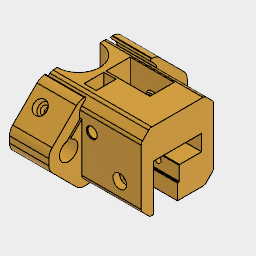
Y_Carriage_1.0_F01 (Autodesk Fusion 360 design; units mm, degrees)
Autodesk Fusion 360 part; units mm, degrees
sketch "スケッチ1" plane through (0, 0, 0) normal (1, 0, 0) x (0, 1, 0)
  line L0 (-17.5, 17.5) -> (17.5, 17.5)
  line L1 (17.5, 17.5) -> (31.5, 3.5)
  line L2 (31.5, 3.5) -> (31.5, -3.5)
  line L3 (31.5, -3.5) -> (17.5, -17.5)
  line L4 (17.5, -17.5) -> (-17.5, -17.5)
  line L5 (-17.5, -17.5) -> (-31.5, -3.5)
  line L6 (-31.5, -3.5) -> (-31.5, 3.5)
  line L7 (-31.5, 3.5) -> (-17.5, 17.5)
  circle A0 centre (-22.5, 0) radius 4.2
  circle A1 centre (22.5, 0) radius 4.2
  line L8 (-12.5, 17.5) -> (-16.5, 13.5)
  line L9 (-16.5, 13.5) -> (-16.5, -13.5)
  line L10 (-16.5, -13.5) -> (-12.5, -17.5)
  line L11 (12.5, 17.5) -> (16.5, 13.5)
  line L12 (16.5, 13.5) -> (16.5, -13.5)
  line L13 (16.5, -13.5) -> (12.5, -17.5)
  line L14 (-13.9142, 17.5) -> (-17.5, 13.9142)
  line L15 (-17.5, 13.9142) -> (-17.5, 9.9071)
  line L16 (-17.5, 9.9071) -> (-23.2802, 4.1269)
  line L17 (-21.8444, 4.1485) -> (-16.5, 9.4929)
  line L18 (-22.5, 0) -> (-22.5, 4.2) construction
  line L19 (-22.5, 4.2) -> (-16.5, 10.2) construction
  line L20 (-22.5, 4.2) -> (-14.0147, 4.2) construction
  line L21 (0, 17.5) -> (0, -17.5) construction
  line L22 (17.5, 9.9071) -> (23.2802, 4.1269)
  line L23 (21.8444, 4.1485) -> (16.5, 9.4929)
  line L24 (17.5, 13.9142) -> (17.5, 9.9071)
  line L25 (13.9142, 17.5) -> (17.5, 13.9142)
  line L26 (12.5, 17.5) -> (16.5, 13.5)
  dimension "d1" = 35
  dimension "d2" = 17.5
  dimension "d3" = 63
  dimension "d4" = 31.5
  dimension "d5" = 14
  dimension "d6" = 14
  dimension "d7" = 14
  dimension "d8" = 14
  dimension "d9" = 14
  dimension "d10" = 14
  dimension "d11" = 14
  dimension "d12" = 14
  dimension "d13" = 8.4
  dimension "d14" = 8.4
  dimension "d15" = 9
  dimension "d16" = 9
  dimension "d17" = 17.5
  dimension "d18" = 17.5
  dimension "d19" = 4
  dimension "d20" = 4
  dimension "d21" = 4
  dimension "d22" = 4
  dimension "d23" = 4
  dimension "d24" = 4
  dimension "d25" = 4
  dimension "d26" = 4
  dimension "d27" = 33
  dimension "d28" = 16.5
  dimension "d29" = 1
  dimension "d30" = 1
  dimension "d31" = 1
  dimension "d32" = 45
  dimension "d33" = 0.5
  measures "d1" distance of L0 L4
  measures "d2" distance of origin L0
  measures "d3" distance of L2 L6
  measures "d4" distance of origin L6
  measures "d5" distance of L0.end L2
  measures "d6" distance of L2.end L3.end
  measures "d7" distance of L0.start L6.end
  measures "d8" distance of L4.end L5.end
  measures "d9" distance of L0.end L1.end
  measures "d10" distance of L2.end L3.end
  measures "d11" distance of L0.start L6.end
  measures "d12" distance of L4.end L5.end
  measures "d13" diameter of A0
  measures "d14" diameter of A1
  measures "d15" distance of L6 A0.centre
  measures "d16" distance of L2 A1.centre
  measures "d17" distance of L0 A0.centre
  measures "d18" distance of L0 A1.centre
  measures "d19" distance of L8.start L8.end
  measures "d20" distance of L11.start L11.end
  measures "d21" distance of L12.end L13.end
  measures "d22" distance of L9.end L10.end
  measures "d23" distance of L8.start L8.end
  measures "d24" distance of L11.start L11.end
  measures "d25" distance of L12.end L13.end
  measures "d26" distance of L9.end L10.end
  measures "d27" distance of L9 L12
  measures "d28" distance of origin L9
  measures "d29" distance of L8 L14
  measures "d30" distance of L9 L15
  measures "d31" distance of L16 L17
  measures "d32" angle of L19 L20
  measures "d33" distance of L17 L19
extrude "押し出し1" add sketch "スケッチ1" along normal blind 45 contours L0 L4 L8 L9 L10 L11 L12 L13 L26
extrude "押し出し2" add sketch "スケッチ1" along normal blind 18 contours L0 L4 L5 L6 L7 A0 L9 L10 L14 L15 L16 L17 | L0 L1 L2 L3 L4 A1 L12 L13 L22 L23 L24 L25
sketch "スケッチ2" plane through (0, 0, 17.5) normal (0, 0, 1) x (-1, 0, 0)
  line L0 (0, -12.5) -> (0, 12.5)
  line L1 (0, 12.5) -> (-45, 12.5)
  line L2 (-45, 12.5) -> (-45, -12.5)
  line L3 (-45, -12.5) -> (0, -12.5)
  line L4 (-12.5, -11) -> (-32.5, -11)
  line L5 (-32.5, -11) -> (-32.5, 0)
  line L6 (-32.5, 0) -> (-12.5, 0)
  line L7 (-12.5, 0) -> (-12.5, -11)
  line L8 (-12.5, 1) -> (-18, 1)
  line L9 (-18, 1) -> (-18, 10)
  line L10 (-18, 10) -> (-12.5, 10)
  line L11 (-12.5, 10) -> (-12.5, 1)
  circle A0 centre (0, 0) radius 9.7
  line L12 (0, -16.5) -> (-45, -16.5)
  line L13 (0, 16.5) -> (-45, 16.5)
  dimension "d38" = 19.4
  dimension "d39" = 32.5
  dimension "d40" = 5.5
  dimension "d41" = 32.5
  dimension "d42" = 20
  dimension "d43" = 11
  dimension "d44" = 9
  dimension "d45" = 5.5
  dimension "d46" = 6.5
  measures "d38" diameter of A0
  measures "d39" distance of L2 L11
  measures "d40" distance of L9 L11
  measures "d41" distance of L2 L7
  measures "d42" distance of L5 L7
  measures "d43" distance of L4 L6
  measures "d44" distance of L8 L10
  measures "d45" distance of L4 L12
  measures "d46" distance of L10 L13
extrude "押し出し3" cut sketch "スケッチ2" against normal up to surface (35 mm away) contours L0 A0 picked at (-3.2243, 0.2416)
sketch "スケッチ3" plane through (45, 0, 0) normal (1, 0, 0) x (0, 1, 0)
  line L0 (-12.5, 17.5) -> (-16.5, 13.5)
  line L1 (-16.5, 13.5) -> (-16.5, -13.5)
  line L2 (-16.5, -13.5) -> (-12.5, -17.5)
  line L3 (-12.5, -17.5) -> (12.5, -17.5)
  line L4 (12.5, -17.5) -> (16.5, -13.5)
  line L5 (16.5, -13.5) -> (16.5, 13.5)
  line L6 (16.5, 13.5) -> (12.5, 17.5)
  line L7 (12.5, 17.5) -> (-12.5, 17.5)
  line L8 (-11, 3.635) -> (0, 3.635)
  line L9 (0, 3.635) -> (0, -17.5)
  line L10 (0, -17.5) -> (-11, -17.5)
  line L11 (-11, -17.5) -> (-11, 3.635)
  line L12 (0, 3.635) -> (11, 3.635)
  line L13 (11, 3.635) -> (11, -3.635)
  line L14 (11, -3.635) -> (0, -3.635)
  line L15 (0, -3.635) -> (0, 3.635)
  dimension "d49" = 5.5
  dimension "d50" = 11
  dimension "d51" = 11
  dimension "d52" = 21.135
  dimension "d53" = 7.27
  measures "d49" distance of L1 L11
  measures "d50" distance of L9 L11
  measures "d51" distance of L9 L13
  measures "d52" distance of L8 L10
  measures "d53" distance of L12 L14
extrude "押し出し4" cut sketch "スケッチ3" against normal blind 19.77 contours L3 L8 L9 L10 L11 L15
fillet "フィレット1" radius 10 1 edges at (25.23, -5.5, 3.635)
extrude "押し出し5" cut sketch "スケッチ2" against normal blind 21.135 contours L4 L5 L6 L7
extrude "押し出し6" cut sketch "スケッチ3" against normal up to surface (12.5 mm away) contours L9 L12 L13 L14 L15
extrude "押し出し7" cut sketch "スケッチ2" against normal up to surface (35 mm away) contours L8 L9 L10 L11
fillet "フィレット2" radius 10 1 edges at (12.5, 5.5, -3.635)
sketch "スケッチ4" plane through (0, 0, 0) normal (0, -1, 0) x (1, 0, 0)
  line L0 (45, -3.635) -> (25.6099, -3.635)
  arc A0 (25.6099, -3.635) -> (25.23, -6.365) centre (35.23, -6.365) ccw
  line L1 (25.23, -6.365) -> (25.23, -17.5)
  line L2 (25.23, -17.5) -> (45, -17.5)
  line L3 (45, -17.5) -> (45, -3.635)
  line L4 (45, -3.635) -> (31, -3.635)
  line L5 (31, -3.635) -> (31, -10.45)
  line L6 (31, -10.45) -> (45, -10.45)
  line L7 (45, -10.45) -> (45, -3.635)
  dimension "d64" = 6.815
  dimension "d65" = 14
  measures "d64" distance of L4 L6
  measures "d65" distance of L5 L7
extrude "押し出し8" cut sketch "スケッチ4" against normal blind 0.8 contours L0 L3 L4 L5 L6 L7
sketch "スケッチ5" plane through (0, -16.5, 0) normal (0, -1, 0) x (1, 0, 0)
  line L0 (0, 9.4929) -> (18, 9.4929)
  line L1 (18, 9.4929) -> (18, -13.5)
  line L2 (18, -13.5) -> (45, -13.5)
  line L3 (45, -13.5) -> (45, 13.5)
  line L4 (45, 13.5) -> (0, 13.5)
  line L5 (0, 13.5) -> (0, 9.4929)
  circle A0 centre (35.23, -6.365) radius 1.5
  circle A1 centre (35.23, -6.365) radius 3.1
  line L6 (18, -17.5) -> (45, -17.5)
  dimension "d68" = 3
  dimension "d69" = 6.2
  dimension "d70" = 9.77
  dimension "d71" = 11.135
  measures "d68" diameter of A0
  measures "d69" diameter of A1
  measures "d70" distance of L3 A0.centre
  measures "d71" distance of A0.centre L6
extrude "押し出し9" cut sketch "スケッチ5" against normal up to surface (33 mm away) contours A0
extrude "押し出し10" cut sketch "スケッチ5" against normal blind 3 contours A1
sketch "スケッチ6" plane through (0, 16.5, 0) normal (0, 1, 0) x (-1, 0, 0)
  circle A0 centre (-35.23, -6.365) radius 1.5
  line L0 (-18, 9.4929) -> (0, 9.4929)
  line L1 (0, 9.4929) -> (0, 13.5)
  line L2 (0, 13.5) -> (-45, 13.5)
  line L3 (-45, 13.5) -> (-45, -13.5)
  line L4 (-45, -13.5) -> (-18, -13.5)
  line L5 (-18, -13.5) -> (-18, 9.4929)
  circle A1 centre (-35.23, -6.365) radius 2.5
  circle A2 centre (-35.23, -6.365) radius 2.25
  circle A3 centre (-22.5, 6.365) radius 1.5
  circle A4 centre (-22.5, 6.365) radius 3.1
  line L6 (0, 17.5) -> (-45, 17.5)
  dimension "d76" = 5
  dimension "d77" = 4.5
  dimension "d82" = 3
  dimension "d83" = 6.2
  dimension "d88" = 11.135
  dimension "d89" = 22.5
  measures "d76" diameter of A1
  measures "d77" diameter of A2
  measures "d82" diameter of A3
  measures "d83" diameter of A4
  measures "d88" distance of A3.centre L6
  measures "d89" distance of L3 A3.centre
extrude "押し出し11" cut sketch "スケッチ6" against normal blind 5 contours A2
extrude "押し出し12" cut sketch "スケッチ6" against normal blind 0.5 contours A1
extrude "押し出し13" cut sketch "スケッチ6" against normal up to surface (33 mm away) contours A3
extrude "押し出し14" cut sketch "スケッチ6" against normal blind 3 contours A4
sketch "スケッチ7" plane through (0, -16.5, 0) normal (0, -1, 0) x (1, 0, 0)
  circle A0 centre (22.5, 6.365) radius 1.5
  circle A1 centre (35.23, -6.365) radius 3.1
  line L0 (0, 9.4929) -> (18, 9.4929)
  line L1 (18, 9.4929) -> (18, -13.5)
  line L2 (18, -13.5) -> (45, -13.5)
  line L3 (45, -13.5) -> (45, 13.5)
  line L4 (45, 13.5) -> (0, 13.5)
  line L5 (0, 13.5) -> (0, 9.4929)
  circle A2 centre (22.5, 6.365) radius 2.5
  circle A3 centre (22.5, 6.365) radius 2.25
  dimension "d90" = 5
  dimension "d91" = 4.5
  measures "d90" diameter of A2
  measures "d91" diameter of A3
extrude "押し出し15" cut sketch "スケッチ7" against normal blind 5 contours A3
extrude "押し出し16" cut sketch "スケッチ7" against normal blind 0.5 contours A2
sketch "スケッチ8" plane through (0, -11, 0) normal (0, 1, 0) x (-1, 0, 0)
  circle A0 centre (-35.23, -6.365) radius 1.5
  arc A1 (-25.23, -6.365) -> (-35.23, 3.635) centre (-35.23, -6.365) ccw
  line L0 (-35.23, 3.635) -> (-45, 3.635)
  line L1 (-45, 3.635) -> (-45, -17.5)
  line L2 (-45, -17.5) -> (-25.23, -17.5)
  line L3 (-25.23, -17.5) -> (-25.23, -6.365)
  circle A2 centre (-35.23, -6.365) radius 2.75
  dimension "d96" = 5.5
  measures "d96" diameter of A2
sketch "スケッチ9" plane through (0, 11, 0) normal (0, -1, 0) x (1, 0, 0)
  circle A0 centre (22.5, 6.365) radius 1.5
  arc A1 (12.5, 6.365) -> (22.5, -3.635) centre (22.5, 6.365) ccw
  line L0 (22.5, -3.635) -> (45, -3.635)
  line L1 (45, -3.635) -> (45, 3.635)
  line L2 (45, 3.635) -> (32.5, 3.635)
  line L3 (32.5, 3.635) -> (32.5, 17.5)
  line L4 (32.5, 17.5) -> (12.5, 17.5)
  line L5 (12.5, 17.5) -> (12.5, 6.365)
  circle A2 centre (22.5, 6.365) radius 2.75
  dimension "d101" = 5.5
  measures "d101" diameter of A2
sketch "スケッチ10" plane through (0, 0, 0) normal (0, 1, 0) x (-1, 0, 0)
  circle A0 centre (-22.5, 6.365) radius 1.5
  arc A1 (-22.5, -3.635) -> (-12.5, 6.365) centre (-22.5, 6.365) ccw
  line L0 (-12.5, 6.365) -> (-12.5, 17.5)
  line L1 (-12.5, 17.5) -> (-32.5, 17.5)
  line L2 (-32.5, 17.5) -> (-32.5, 3.635)
  line L3 (-32.5, 3.635) -> (-35.23, 3.635)
  arc A2 (-25.6099, -3.635) -> (-35.23, 3.635) centre (-35.23, -6.365) ccw
  line L4 (-25.6099, -3.635) -> (-22.5, -3.635)
  circle A3 centre (-22.5, 6.365) radius 2.75
  dimension "d102" = 5.5
  measures "d102" diameter of A3
extrude "押し出し17" add sketch "スケッチ8" along normal blind 0.8 draft -30 contours A0 | A2
extrude "押し出し18" add sketch "スケッチ10" along normal blind 0.8 draft -30 contours A0 | A3
extrude "押し出し19" add sketch "スケッチ9" along normal blind 0.8 draft -30 contours A0 | A2
extrude "押し出し20" cut 1 faces at (22.2707, 11, 7.4522) along direction (0, -1, 0) up to surface (0.8 mm away)
extrude "押し出し21" cut 1 faces at (22.3547, 0, 7.329) along direction (0, 1, 0) up to surface (0.8 mm away)
extrude "押し出し22" cut 1 faces at (34.8579, -11, -6.0994) along direction (0, 1, 0) up to surface (0.8 mm away)
sketch "スケッチ11" plane through (0, -17.5, 17.5) normal (0, -0.707107, 0.707107) x (1, 0, 0)
  line L0 (0, 0) -> (0, -19.799)
  line L1 (0, -19.799) -> (18, -19.799)
  line L2 (18, -19.799) -> (18, 0)
  line L3 (18, 0) -> (0, 0)
  circle A0 centre (6, -8.4099) radius 3
  circle A1 centre (6, -8.4099) radius 1.75
  line L4 (0, -24.7487) -> (18, -24.7487)
  line L5 (3, -10.142) -> (6, -11.874)
  line L6 (6, -11.874) -> (9, -10.142)
  line L7 (9, -10.142) -> (9, -6.6779)
  line L8 (9, -6.6779) -> (6, -4.9458)
  line L9 (6, -4.9458) -> (3, -6.6779)
  line L10 (3, -6.6779) -> (3, -10.142)
  point P0 (6, -8.4099)
  dimension "d113" = 6
  dimension "d114" = 3.5
  dimension "d115" = 16.3388
  dimension "d116" = 6
  dimension "d132" = 3
  measures "d113" diameter of A0
  measures "d114" diameter of A1
  measures "d115" distance of P0 L4
  measures "d116" distance of L0 P0
  measures "d132" distance of P0 L9
extrude "押し出し23" cut sketch "スケッチ11" against normal blind 30 contours A1
extrude "押し出し24" cut sketch "スケッチ11" against normal blind 3 contours A0
sketch "スケッチ12" plane through (0, 17.5, 17.5) normal (0, 0.707107, 0.707107) x (-1, 0, 0)
  line L0 (0, -19.799) -> (0, 0)
  line L1 (0, 0) -> (-18, 0)
  line L2 (-18, 0) -> (-18, -19.799)
  line L3 (-18, -19.799) -> (0, -19.799)
  circle A0 centre (-6, -8.4099) radius 3
  circle A1 centre (-6, -8.4099) radius 1.75
  line L4 (0, -24.7487) -> (-18, -24.7487)
  line L5 (-3, -6.6779) -> (-6, -4.9458)
  line L6 (-6, -4.9458) -> (-9, -6.6779)
  line L7 (-9, -6.6779) -> (-9, -10.142)
  line L8 (-9, -10.142) -> (-6, -11.874)
  line L9 (-6, -11.874) -> (-3, -10.142)
  line L10 (-3, -10.142) -> (-3, -6.6779)
  point P0 (-6, -8.4099)
  dimension "d121" = 6
  dimension "d122" = 3.5
  dimension "d123" = 6
  dimension "d124" = 16.3388
  dimension "d136" = 3
  measures "d121" diameter of A0
  measures "d122" diameter of A1
  measures "d123" distance of L0 P0
  measures "d124" distance of P0 L4
  measures "d136" distance of P0 L5
extrude "押し出し25" cut sketch "スケッチ12" against normal blind 30 contours A1
extrude "押し出し26" cut sketch "スケッチ12" against normal blind 3 contours A0
extrude "押し出し27" cut sketch "スケッチ11" against normal blind 15 from surface at -15 contours A0 | A0 L6 L7 | A0 L7 L8 | A0 L8 L9 | A0 L5 L6 | A0 L9 L10 | A0 L5 L10 | A1
extrude "押し出し28" cut sketch "スケッチ12" against normal blind 15 from surface at -15 contours A0 | A0 L9 L10 | A0 L5 L10 | A0 L5 L6 | A0 L8 L9 | A0 L6 L7 | A0 L7 L8 | A1
sketch "スケッチ14" plane through (0, 0, 0) normal (1, 0, 0) x (0, 1, 0)
  circle A0 centre (12.5, 12.5) radius 2.5
  circle A1 centre (12.5, 12.5) radius 2.35
  circle A2 centre (12.5, 12.5) radius 1.6
  dimension "d140" = 5
  dimension "d141" = 4.7
  dimension "d142" = 3.2
  dimension "d143" = 12.5
  dimension "d144" = 12.5
  measures "d140" diameter of A0
  measures "d141" diameter of A1
  measures "d142" diameter of A2
  measures "d143" distance of origin A0.centre
  measures "d144" distance of origin A0.centre
extrude "押し出し29" cut sketch "スケッチ14" along normal blind 10 contours A2
extrude "押し出し30" cut sketch "スケッチ14" along normal blind 5 contours A1
extrude "押し出し31" cut sketch "スケッチ14" along normal blind 0.5 contours A0
pattern_circular "C パターン1" count 4 over 360 about axis through (1.75, 0, 0) along (1, 0, 0) of "押し出し29", "押し出し30", "押し出し31"
fillet "フィレット3" radius 5 8 edges at (9, 17.5, -17.5) (9, 31.5, -3.5) (9, 31.5, 3.5) (9, 17.5, 17.5) (9, -17.5, 17.5) (9, -31.5, 3.5) (9, -31.5, -3.5) (9, -17.5, -17.5)
fillet "フィレット4" radius 2 8 edges at (31.5, 12.5, -17.5) (31.5, 16.5, -13.5) (22.5, 16.5, 13.5) (22.5, 12.5, 17.5) (22.5, -12.5, 17.5) (22.5, -16.5, 13.5) (31.5, -16.5, -13.5) (31.5, -12.5, -17.5)
fillet "フィレット5" radius 3 2 edges at (9, 17.5, 13.9142) (9, -17.5, 13.9142)
fillet "フィレット6" radius 0.5 6 edges at (9, 13.9142, 17.5) (9, -13.9142, 17.5) (9, 21.8444, 4.1485) (9, 23.2802, 4.1269) (9, -23.2802, 4.1269) (9, -21.8444, 4.1485)
fillet "フィレット7" radius 0.2 2 edges at (38, 0.8, -3.635) (38, 0.8, -10.45)
equation "d2 = d1 / 2"
equation "d4 = d3 / 2"
equation "d9 = d5"
equation "d10 = d6"
equation "d11 = d7"
equation "d12 = d8"
equation "d17 = d2"
equation "d18 = d2"
equation "d23 = d19"
equation "d24 = d20"
equation "d25 = d21"
equation "d26 = d22"
equation "d28 = d27 / 2"
equation "d33 = d31 / 2"
equation "d41 = d39"
